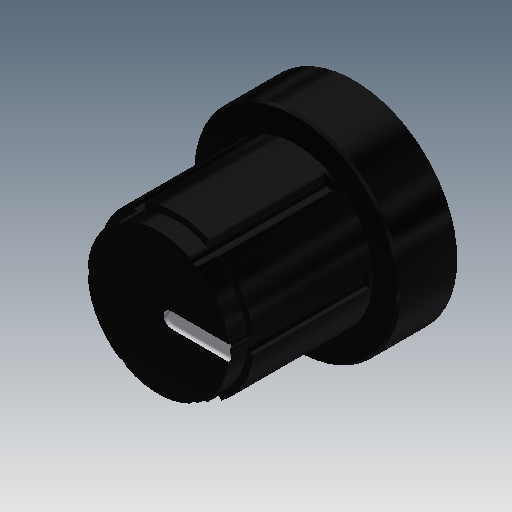
# Autodesk Inventor part: Potentiometer knob
Saved by Autodesk Inventor 2017 (Build 210142000, 142)
## iProperties
Created: 2017-01-24
Part Number: Potentiometer knob
Material: PC/ABS Plastic
Document SubType Name: Modeling
Designer: Miguel Grassi
Density: 0.357273 g/cm^3
Appearance: Glossy - Black
Author: Miguel Grassi
Autodesk Inventor part; units mm, degrees
ref_plane "YZ Plane" through (0, 0, 0) normal (1, 0, 0) x (0, 1, 0)
ref_plane "XZ Plane" through (0, 0, 0) normal (0, 1, 0) x (-1, 0, 0)
ref_plane "XY Plane" through (0, 0, 0) normal (0, 0, 1) x (1, 0, 0)
sketch "Sketch1" plane through (0, 0, 0) normal (0, 0, 1) x (1, 0, 0)
  circle A0 centre (0, 0) radius 9.5
  circle A1 centre (0, 0) radius 7.1
  dimension "d0" = 19
  dimension "d1" = 14.2
  constraints: 2 centre point, 2 coincident
  measures "d0" diameter of A0
  measures "d1" diameter of A1
extrude "Extrusion1" add sketch "Sketch1" along normal blind 12.6 contours A1
extrude "Extrusion2" add sketch "Sketch1" against normal blind 5.35
hole "Hole1" at (0, 0, 0) direction (0, 0, 1) diameter 6 depth 10
sketch "Sketch2" plane through (0, 0, 12.6) normal (0, 0, 1) x (1, 0, 0)
  arc A0 (7.065241, 0.698467) -> (7.065335, -0.700746) centre (7.041831, -0.001141) ccw
  arc A1 (7.065335, -0.700746) -> (7.065241, 0.698467) centre (1.208445, -0.001533) ccw
  arc A2 (1.208445, 0.698467) -> (1.208539, -0.701533) centre (1.208445, -0.001533) ccw
  line L0 (1.208445, 0.698467) -> (7.065241, 0.698467)
  circle A3 centre (0, 0) radius 7.1
  line L1 (7.065335, -0.700746) -> (1.208539, -0.701533)
  dimension "d25" = 0.7
  dimension "d26" = 0.7
  constraints: 6 point on circle, 4 end point, 3 centre point, 2 coincident, 2 tangent, 1 horizontal, 2 other
  measures "d25" radius of A0
  measures "d26" radius of A2
sketch "Sketch2 outline for Extrusion3" plane through (0, 0, 12.6) normal (0, 0, 1) x (1, 0, 0)
  arc A0 (7.065241, 0.698467) -> (7.065335, -0.700746) centre (7.041831, -0.001141) ccw
  arc A1 (7.065335, -0.700746) -> (7.065241, 0.698467) centre (1.208445, -0.001533) ccw
extrude "Extrusion3" cut sketch "Sketch2 outline for Extrusion3" against normal blind 12.3
pattern_circular "Circular Pattern1" count 6 over 360 about axis through (0, 0, 0) along (0, 0, 1) of "Extrusion3"
sketch "Sketch3" plane through (0, 0, 12.6) normal (0, 0, 1) x (1, 0, 0)
  circle A0 centre (0, 0) radius 6.488045
  circle A1 centre (0, 0) radius 7.1
  constraints: 2 centre point, 2 coincident
extrude "Extrusion4" cut sketch "Sketch3" against normal blind 1.65
sketch "Sketch2 outline for Extrusion5" plane through (0, 0, 12.6) normal (0, 0, 1) x (1, 0, 0)
  line L0 (7.065241, 0.698467) -> (1.208445, 0.698467)
  arc A0 (7.065335, -0.700746) -> (7.065241, 0.698467) centre (1.208445, -0.001533) ccw
  line L1 (1.208539, -0.701533) -> (7.065335, -0.700746)
  arc A1 (1.208445, 0.698467) -> (1.208539, -0.701533) centre (1.208445, -0.001533) ccw
extrude "Extrusion5" cut sketch "Sketch2 outline for Extrusion5" against normal blind 0.25
fillet "Fillet1" radius 0.25 3 edges at (0.5084, -0.0016, 12.35) (3.8293, -0.7012, 12.35) (3.8294, 0.6985, 12.35)
chamfer "Chamfer1" distance 0.2 angle 45 1 edges at (-9.5, 0, 0)
equation "\"d26\" = d25"
body "Solid1"
